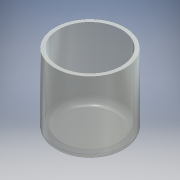
# Autodesk Inventor part: vaso
Saved by Autodesk Inventor 2016 (Build 200138000, 138)
## iProperties
Created: 2016-09-14
Part Number: vaso
Material: Vidrio
Document SubType Name: Modeling
Designer: Isabel
Density: 2.18 g/cm^3
Appearance: Claro
Author: Isabel
Autodesk Inventor part; units mm, degrees
ref_plane "YZ Plane" through (0, 0, 0) normal (1, 0, 0) x (0, 1, 0)
ref_plane "XZ Plane" through (0, 0, 0) normal (0, 1, 0) x (-1, 0, 0)
ref_plane "XY Plane" through (0, 0, 0) normal (0, 0, 1) x (1, 0, 0)
sketch "Boceto2" plane through (0, 0, 0) normal (0, 0, 1) x (1, 0, 0)
  line L0 (0, 0) -> (40, 0)
  line L1 (48, 8) -> (48, 100)
  line L2 (48, 100) -> (43, 100)
  line L3 (43, 100) -> (43, 15)
  line L4 (33, 5) -> (0, 5)
  line L5 (0, 5) -> (0, 0)
  arc A0 (33, 5) -> (43, 15) centre (33, 15) ccw
  arc A1 (40, 0) -> (48, 8) centre (40, 8) ccw
  point P0 (48, 0)
  point P1 (43, 5)
  dimension "d4" = 5
  dimension "d5" = 100
  dimension "d6" = 5
  dimension "d7" = 48
  dimension "d9" = 10
  dimension "d10" = 8
  constraints: 12 end point, 5 perpendicular, 4 point on circle, 4 point on line, 4 tangent, 2 centre point, 1 horizontal
  measures "d4" distance between parallel lines of L1 L3
  measures "d5" distance between parallel lines of L0 L2
  measures "d6" distance between parallel lines of L4 L0
  measures "d7" distance between parallel lines of L1 L5
  measures "d9" radius of A0
  measures "d10" radius of A1
revolve "Revolución1" add sketch "Boceto2" angle 360 about axis through (0, 5, 0) along (0, -1, 0)
move or copy body "Desplazar cuerpo1" bodies to move or copy 1 copy no rotation origin (0, 0, 0) rotation axis (1, 0, 0) rotation angle 90
